Autodesk Inventor part; units mm, degrees
(part 2 of 2)
  line L284 (-20.2182, -37.2019) -> (-20.2182, -36.6708)
  line L285 (-20.2182, -36.6708) -> (-19.576, -36.6708)
  line L286 (-19.576, -36.6708) -> (-19.576, -35.0579)
  line L287 (-19.576, -35.0579) -> (-20.2182, -35.0579)
  line L288 (-20.2182, -35.0579) -> (-20.2182, -34.5614)
  spline S239 degree 2 poles (-20.2182, -34.5614) (-20.0774, -34.5614) (-19.7983, -34.5244) (-19.7143, -34.4848) knots 0 0 0 1 2 2 2
  spline S240 degree 2 poles (-19.7143, -34.4848) (-19.6179, -34.4354) (-19.5093, -34.27) (-19.4994, -34.1465) knots 0 0 0 1 2 2 2
  line L289 (-19.4994, -34.1465) -> (-18.8325, -34.1465)
  line L290 (-18.8325, -34.1465) -> (-18.8325, -36.6708)
  line L291 (-18.8325, -36.6708) -> (-18.2051, -36.6708)
  line L292 (-18.2051, -36.6708) -> (-18.2051, -37.2019)
  spline S241 degree 2 poles (-15.4164, -36.1645) (-15.4164, -36.6461) (-16.0265, -37.2661) (-16.5601, -37.2661) knots 0 0 0 1 2 2 2
  spline S242 degree 2 poles (-16.5601, -37.2661) (-16.8268, -37.2661) (-17.2443, -37.1129) (-17.39, -36.9623) knots 0 0 0 1 2 2 2
  spline S243 degree 2 poles (-17.39, -36.9623) (-17.5629, -36.7869) (-17.7481, -36.2312) (-17.7481, -35.8434) knots 0 0 0 1 2 2 2
  spline S244 degree 2 poles (-17.7481, -35.8434) (-17.7481, -35.4432) (-17.5752, -34.8208) (-17.3801, -34.5812) knots 0 0 0 1 2 2 2
  spline S245 degree 2 poles (-17.3801, -34.5812) (-17.1949, -34.3539) (-16.5922, -34.0971) (-16.1797, -34.0971) knots 0 0 0 1 2 2 2
  spline S246 degree 2 poles (-16.1797, -34.0971) (-16.029, -34.0971) (-15.7277, -34.1366) (-15.6733, -34.1489) knots 0 0 0 1 2 2 2
  line L293 (-15.6733, -34.1489) -> (-15.6733, -34.7467)
  line L294 (-15.6733, -34.7467) -> (-15.7277, -34.7467)
  spline S247 degree 2 poles (-15.7277, -34.7467) (-15.782, -34.7195) (-16.029, -34.6528) (-16.1871, -34.6528) knots 0 0 0 1 2 2 2
  spline S248 degree 2 poles (-16.1871, -34.6528) (-16.5452, -34.6528) (-16.9355, -35.0307) (-16.9824, -35.3815) knots 0 0 0 1 2 2 2
  spline S249 degree 2 poles (-16.9824, -35.3815) (-16.8318, -35.2851) (-16.523, -35.1715) (-16.3279, -35.1715) knots 0 0 0 1 2 2 2
  spline S250 degree 2 poles (-16.3279, -35.1715) (-16.1624, -35.1715) (-15.8734, -35.2604) (-15.7623, -35.3444) knots 0 0 0 1 2 2 2
  spline S251 degree 2 poles (-15.7623, -35.3444) (-15.6042, -35.4654) (-15.4164, -35.8582) (-15.4164, -36.1645) knots 0 0 0 1 2 2 2
  spline S252 degree 2 poles (-16.3081, -36.6239) (-16.2488, -36.5498) (-16.1846, -36.3769) (-16.1846, -36.2015) knots 0 0 0 1 2 2 2
  spline S253 degree 2 poles (-16.1846, -36.2015) (-16.1846, -36.0533) (-16.2587, -35.8606) (-16.3254, -35.8038) knots 0 0 0 1 2 2 2
  spline S254 degree 2 poles (-16.3254, -35.8038) (-16.3946, -35.7446) (-16.565, -35.7026) (-16.6613, -35.7026) knots 0 0 0 1 2 2 2
  spline S255 degree 2 poles (-16.6613, -35.7026) (-16.7428, -35.7026) (-16.9108, -35.7446) (-16.9849, -35.7742) knots 0 0 0 1 2 2 2
  spline S256 degree 2 poles (-16.9849, -35.7742) (-16.9849, -35.794) (-16.9899, -35.8878) (-16.9899, -35.9594) knots 0 0 0 1 2 2 2
  spline S257 degree 2 poles (-16.9899, -35.9594) (-16.9899, -36.2237) (-16.8985, -36.5424) (-16.8268, -36.6239) knots 0 0 0 1 2 2 2
  spline S258 degree 2 poles (-16.8268, -36.6239) (-16.775, -36.6906) (-16.6366, -36.7474) (-16.5625, -36.7474) knots 0 0 0 1 2 2 2
  spline S259 degree 2 poles (-16.5625, -36.7474) (-16.5008, -36.7474) (-16.3575, -36.6856) (-16.3081, -36.6239) knots 0 0 0 1 2 2 2
  line L295 (-13.0601, -37.2019) -> (-13.7764, -37.2019)
  line L296 (-13.7764, -37.2019) -> (-13.7764, -34.9023)
  line L297 (-13.7764, -34.9023) -> (-13.0601, -34.9023)
  line L298 (-13.0601, -34.9023) -> (-13.0601, -37.2019)
  line L299 (-13.0378, -34.5738) -> (-13.7961, -34.5738)
  line L300 (-13.7961, -34.5738) -> (-13.7961, -34.0155)
  line L301 (-13.7961, -34.0155) -> (-13.0378, -34.0155)
  line L302 (-13.0378, -34.0155) -> (-13.0378, -34.5738)
  line L303 (-10.3603, -37.2019) -> (-11.0816, -37.2019)
  line L304 (-11.0816, -37.2019) -> (-11.0816, -36.0632)
  spline S260 degree 2 poles (-11.0816, -36.0632) (-11.0816, -35.9224) (-11.1038, -35.6458) (-11.1334, -35.5815) knots 0 0 0 1 2 2 2
  spline S261 degree 2 poles (-11.1334, -35.5815) (-11.1705, -35.5025) (-11.3088, -35.4358) (-11.4274, -35.4358) knots 0 0 0 1 2 2 2
  spline S262 degree 2 poles (-11.4274, -35.4358) (-11.5138, -35.4358) (-11.6941, -35.5025) (-11.7954, -35.5741) knots 0 0 0 1 2 2 2
  line L305 (-11.7954, -35.5741) -> (-11.7954, -37.2019)
  line L306 (-11.7954, -37.2019) -> (-12.5117, -37.2019)
  line L307 (-12.5117, -37.2019) -> (-12.5117, -34.9023)
  line L308 (-12.5117, -34.9023) -> (-11.7954, -34.9023)
  line L309 (-11.7954, -34.9023) -> (-11.7954, -35.1567)
  spline S263 degree 2 poles (-11.7954, -35.1567) (-11.62, -35.0085) (-11.2866, -34.8405) (-11.084, -34.8405) knots 0 0 0 1 2 2 2
  spline S264 degree 2 poles (-11.084, -34.8405) (-10.7333, -34.8405) (-10.3603, -35.2851) (-10.3603, -35.705) knots 0 0 0 1 2 2 2
  line L310 (-10.3603, -35.705) -> (-10.3603, -37.2019)
  spline S265 degree 2 poles (-8.7029, -37.2636) (-8.987, -37.2636) (-9.4588, -37.1204) (-9.6341, -36.9722) knots 0 0 0 1 2 2 2
  spline S266 degree 2 poles (-9.6341, -36.9722) (-9.8046, -36.8215) (-9.9972, -36.3695) (-9.9972, -36.0632) knots 0 0 0 1 2 2 2
  spline S267 degree 2 poles (-9.9972, -36.0632) (-9.9972, -35.7322) (-9.7898, -35.2703) (-9.6094, -35.1221) knots 0 0 0 1 2 2 2
  spline S268 degree 2 poles (-9.6094, -35.1221) (-9.439, -34.9789) (-8.9746, -34.8405) (-8.7227, -34.8405) knots 0 0 0 1 2 2 2
  spline S269 degree 2 poles (-8.7227, -34.8405) (-8.5325, -34.8405) (-8.1521, -34.9295) (-7.9595, -35.0258) knots 0 0 0 1 2 2 2
  line L311 (-7.9595, -35.0258) -> (-7.9595, -35.6383)
  line L312 (-7.9595, -35.6383) -> (-8.0509, -35.6383)
  spline S270 degree 2 poles (-8.0509, -35.6383) (-8.0953, -35.5964) (-8.2188, -35.4976) (-8.2929, -35.458) knots 0 0 0 1 2 2 2
  spline S271 degree 2 poles (-8.2929, -35.458) (-8.372, -35.4136) (-8.5671, -35.3543) (-8.6881, -35.3543) knots 0 0 0 1 2 2 2
  spline S272 degree 2 poles (-8.6881, -35.3543) (-8.9623, -35.3543) (-9.2636, -35.7371) (-9.2636, -36.0632) knots 0 0 0 1 2 2 2
  spline S273 degree 2 poles (-9.2636, -36.0632) (-9.2636, -36.409) (-8.9425, -36.7499) (-8.6758, -36.7499) knots 0 0 0 1 2 2 2
  spline S274 degree 2 poles (-8.6758, -36.7499) (-8.5399, -36.7499) (-8.3374, -36.6881) (-8.2633, -36.6436) knots 0 0 0 1 2 2 2
  spline S275 degree 2 poles (-8.2633, -36.6436) (-8.1917, -36.6017) (-8.0879, -36.5078) (-8.0509, -36.4707) knots 0 0 0 1 2 2 2
  line L313 (-8.0509, -36.4707) -> (-7.9595, -36.4707)
  line L314 (-7.9595, -36.4707) -> (-7.9595, -37.0858)
  spline S276 degree 2 poles (-7.9595, -37.0858) (-8.0212, -37.1129) (-8.1818, -37.1821) (-8.2658, -37.2043) knots 0 0 0 1 2 2 2
  spline S277 degree 2 poles (-8.2658, -37.2043) (-8.3695, -37.234) (-8.5523, -37.2636) (-8.7029, -37.2636) knots 0 0 0 1 2 2 2
  line L315 (-5.4672, -37.2019) -> (-6.1885, -37.2019)
  line L316 (-6.1885, -37.2019) -> (-6.1885, -36.0632)
  spline S278 degree 2 poles (-6.1885, -36.0632) (-6.1885, -35.9224) (-6.2107, -35.6458) (-6.2403, -35.5815) knots 0 0 0 1 2 2 2
  spline S279 degree 2 poles (-6.2403, -35.5815) (-6.2774, -35.5025) (-6.4157, -35.4358) (-6.5343, -35.4358) knots 0 0 0 1 2 2 2
  spline S280 degree 2 poles (-6.5343, -35.4358) (-6.6207, -35.4358) (-6.801, -35.5025) (-6.9023, -35.5741) knots 0 0 0 1 2 2 2
  line L317 (-6.9023, -35.5741) -> (-6.9023, -37.2019)
  line L318 (-6.9023, -37.2019) -> (-7.6186, -37.2019)
  line L319 (-7.6186, -37.2019) -> (-7.6186, -34.018)
  line L320 (-7.6186, -34.018) -> (-6.9023, -34.018)
  line L321 (-6.9023, -34.018) -> (-6.9023, -35.1567)
  spline S281 degree 2 poles (-6.9023, -35.1567) (-6.7269, -35.0085) (-6.3935, -34.8405) (-6.1909, -34.8405) knots 0 0 0 1 2 2 2
  spline S282 degree 2 poles (-6.1909, -34.8405) (-5.8402, -34.8405) (-5.4672, -35.2851) (-5.4672, -35.705) knots 0 0 0 1 2 2 2
  line L322 (-5.4672, -35.705) -> (-5.4672, -37.2019)
  line L323 (6.2592, -34.759) -> (4.9575, -37.2019)
  line L324 (4.9575, -37.2019) -> (4.1078, -37.2019)
  line L325 (4.1078, -37.2019) -> (5.4687, -34.7294)
  line L326 (5.4687, -34.7294) -> (4.0164, -34.7294)
  line L327 (4.0164, -34.7294) -> (4.0164, -34.1539)
  line L328 (4.0164, -34.1539) -> (6.2592, -34.1539)
  line L329 (6.2592, -34.1539) -> (6.2592, -34.759)
  line L330 (8.4896, -34.018) -> (7.2768, -37.8638)
  line L331 (7.2768, -37.8638) -> (6.6889, -37.8638)
  line L332 (6.6889, -37.8638) -> (7.8992, -34.018)
  line L333 (7.8992, -34.018) -> (8.4896, -34.018)
  spline S283 degree 2 poles (11.3968, -36.1645) (11.3968, -36.6461) (10.7867, -37.2661) (10.2532, -37.2661) knots 0 0 0 1 2 2 2
  spline S284 degree 2 poles (10.2532, -37.2661) (9.9864, -37.2661) (9.569, -37.1129) (9.4232, -36.9623) knots 0 0 0 1 2 2 2
  spline S285 degree 2 poles (9.4232, -36.9623) (9.2503, -36.7869) (9.0651, -36.2312) (9.0651, -35.8434) knots 0 0 0 1 2 2 2
  spline S286 degree 2 poles (9.0651, -35.8434) (9.0651, -35.4432) (9.238, -34.8208) (9.4331, -34.5812) knots 0 0 0 1 2 2 2
  spline S287 degree 2 poles (9.4331, -34.5812) (9.6184, -34.3539) (10.2211, -34.0971) (10.6336, -34.0971) knots 0 0 0 1 2 2 2
  spline S288 degree 2 poles (10.6336, -34.0971) (10.7842, -34.0971) (11.0856, -34.1366) (11.1399, -34.1489) knots 0 0 0 1 2 2 2
  line L334 (11.1399, -34.1489) -> (11.1399, -34.7467)
  line L335 (11.1399, -34.7467) -> (11.0856, -34.7467)
  spline S289 degree 2 poles (11.0856, -34.7467) (11.0312, -34.7195) (10.7842, -34.6528) (10.6261, -34.6528) knots 0 0 0 1 2 2 2
  spline S290 degree 2 poles (10.6261, -34.6528) (10.268, -34.6528) (9.8777, -35.0307) (9.8308, -35.3815) knots 0 0 0 1 2 2 2
  spline S291 degree 2 poles (9.8308, -35.3815) (9.9815, -35.2851) (10.2902, -35.1715) (10.4854, -35.1715) knots 0 0 0 1 2 2 2
  spline S292 degree 2 poles (10.4854, -35.1715) (10.6508, -35.1715) (10.9398, -35.2604) (11.051, -35.3444) knots 0 0 0 1 2 2 2
  spline S293 degree 2 poles (11.051, -35.3444) (11.2091, -35.4654) (11.3968, -35.8582) (11.3968, -36.1645) knots 0 0 0 1 2 2 2
  spline S294 degree 2 poles (10.5051, -36.6239) (10.5644, -36.5498) (10.6286, -36.3769) (10.6286, -36.2015) knots 0 0 0 1 2 2 2
  spline S295 degree 2 poles (10.6286, -36.2015) (10.6286, -36.0533) (10.5545, -35.8606) (10.4878, -35.8038) knots 0 0 0 1 2 2 2
  spline S296 degree 2 poles (10.4878, -35.8038) (10.4187, -35.7446) (10.2482, -35.7026) (10.1519, -35.7026) knots 0 0 0 1 2 2 2
  spline S297 degree 2 poles (10.1519, -35.7026) (10.0704, -35.7026) (9.9024, -35.7446) (9.8283, -35.7742) knots 0 0 0 1 2 2 2
  spline S298 degree 2 poles (9.8283, -35.7742) (9.8283, -35.794) (9.8234, -35.8878) (9.8234, -35.9594) knots 0 0 0 1 2 2 2
  spline S299 degree 2 poles (9.8234, -35.9594) (9.8234, -36.2237) (9.9148, -36.5424) (9.9864, -36.6239) knots 0 0 0 1 2 2 2
  spline S300 degree 2 poles (9.9864, -36.6239) (10.0383, -36.6906) (10.1766, -36.7474) (10.2507, -36.7474) knots 0 0 0 1 2 2 2
  spline S301 degree 2 poles (10.2507, -36.7474) (10.3124, -36.7474) (10.4557, -36.6856) (10.5051, -36.6239) knots 0 0 0 1 2 2 2
  line L336 (13.7532, -37.2019) -> (13.0369, -37.2019)
  line L337 (13.0369, -37.2019) -> (13.0369, -34.9023)
  line L338 (13.0369, -34.9023) -> (13.7532, -34.9023)
  line L339 (13.7532, -34.9023) -> (13.7532, -37.2019)
  line L340 (13.7754, -34.5738) -> (13.0171, -34.5738)
  line L341 (13.0171, -34.5738) -> (13.0171, -34.0155)
  line L342 (13.0171, -34.0155) -> (13.7754, -34.0155)
  line L343 (13.7754, -34.0155) -> (13.7754, -34.5738)
  line L344 (16.4529, -37.2019) -> (15.7317, -37.2019)
  line L345 (15.7317, -37.2019) -> (15.7317, -36.0632)
  spline S302 degree 2 poles (15.7317, -36.0632) (15.7317, -35.9224) (15.7094, -35.6458) (15.6798, -35.5815) knots 0 0 0 1 2 2 2
  spline S303 degree 2 poles (15.6798, -35.5815) (15.6427, -35.5025) (15.5044, -35.4358) (15.3859, -35.4358) knots 0 0 0 1 2 2 2
  spline S304 degree 2 poles (15.3859, -35.4358) (15.2994, -35.4358) (15.1191, -35.5025) (15.0178, -35.5741) knots 0 0 0 1 2 2 2
  line L346 (15.0178, -35.5741) -> (15.0178, -37.2019)
  line L347 (15.0178, -37.2019) -> (14.3015, -37.2019)
  line L348 (14.3015, -37.2019) -> (14.3015, -34.9023)
  line L349 (14.3015, -34.9023) -> (15.0178, -34.9023)
  line L350 (15.0178, -34.9023) -> (15.0178, -35.1567)
  spline S305 degree 2 poles (15.0178, -35.1567) (15.1932, -35.0085) (15.5267, -34.8405) (15.7292, -34.8405) knots 0 0 0 1 2 2 2
  spline S306 degree 2 poles (15.7292, -34.8405) (16.0799, -34.8405) (16.4529, -35.2851) (16.4529, -35.705) knots 0 0 0 1 2 2 2
  line L351 (16.4529, -35.705) -> (16.4529, -37.2019)
  spline S307 degree 2 poles (18.1103, -37.2636) (17.8262, -37.2636) (17.3545, -37.1204) (17.1791, -36.9722) knots 0 0 0 1 2 2 2
  spline S308 degree 2 poles (17.1791, -36.9722) (17.0087, -36.8215) (16.816, -36.3695) (16.816, -36.0632) knots 0 0 0 1 2 2 2
  spline S309 degree 2 poles (16.816, -36.0632) (16.816, -35.7322) (17.0235, -35.2703) (17.2038, -35.1221) knots 0 0 0 1 2 2 2
  spline S310 degree 2 poles (17.2038, -35.1221) (17.3742, -34.9789) (17.8386, -34.8405) (18.0905, -34.8405) knots 0 0 0 1 2 2 2
  spline S311 degree 2 poles (18.0905, -34.8405) (18.2807, -34.8405) (18.6611, -34.9295) (18.8538, -35.0258) knots 0 0 0 1 2 2 2
  line L352 (18.8538, -35.0258) -> (18.8538, -35.6383)
  line L353 (18.8538, -35.6383) -> (18.7624, -35.6383)
  spline S312 degree 2 poles (18.7624, -35.6383) (18.7179, -35.5964) (18.5944, -35.4976) (18.5203, -35.458) knots 0 0 0 1 2 2 2
  spline S313 degree 2 poles (18.5203, -35.458) (18.4413, -35.4136) (18.2461, -35.3543) (18.1251, -35.3543) knots 0 0 0 1 2 2 2
  spline S314 degree 2 poles (18.1251, -35.3543) (17.8509, -35.3543) (17.5496, -35.7371) (17.5496, -36.0632) knots 0 0 0 1 2 2 2
  spline S315 degree 2 poles (17.5496, -36.0632) (17.5496, -36.409) (17.8707, -36.7499) (18.1375, -36.7499) knots 0 0 0 1 2 2 2
  spline S316 degree 2 poles (18.1375, -36.7499) (18.2733, -36.7499) (18.4759, -36.6881) (18.55, -36.6436) knots 0 0 0 1 2 2 2
  spline S317 degree 2 poles (18.55, -36.6436) (18.6216, -36.6017) (18.7253, -36.5078) (18.7624, -36.4707) knots 0 0 0 1 2 2 2
  line L354 (18.7624, -36.4707) -> (18.8538, -36.4707)
  line L355 (18.8538, -36.4707) -> (18.8538, -37.0858)
  spline S318 degree 2 poles (18.8538, -37.0858) (18.792, -37.1129) (18.6315, -37.1821) (18.5475, -37.2043) knots 0 0 0 1 2 2 2
  spline S319 degree 2 poles (18.5475, -37.2043) (18.4437, -37.234) (18.261, -37.2636) (18.1103, -37.2636) knots 0 0 0 1 2 2 2
  line L356 (21.346, -37.2019) -> (20.6248, -37.2019)
  line L357 (20.6248, -37.2019) -> (20.6248, -36.0632)
  spline S320 degree 2 poles (20.6248, -36.0632) (20.6248, -35.9224) (20.6025, -35.6458) (20.5729, -35.5815) knots 0 0 0 1 2 2 2
  spline S321 degree 2 poles (20.5729, -35.5815) (20.5358, -35.5025) (20.3975, -35.4358) (20.279, -35.4358) knots 0 0 0 1 2 2 2
  spline S322 degree 2 poles (20.279, -35.4358) (20.1925, -35.4358) (20.0122, -35.5025) (19.9109, -35.5741) knots 0 0 0 1 2 2 2
  line L358 (19.9109, -35.5741) -> (19.9109, -37.2019)
  line L359 (19.9109, -37.2019) -> (19.1946, -37.2019)
  line L360 (19.1946, -37.2019) -> (19.1946, -34.018)
  line L361 (19.1946, -34.018) -> (19.9109, -34.018)
  line L362 (19.9109, -34.018) -> (19.9109, -35.1567)
  spline S323 degree 2 poles (19.9109, -35.1567) (20.0863, -35.0085) (20.4198, -34.8405) (20.6223, -34.8405) knots 0 0 0 1 2 2 2
  spline S324 degree 2 poles (20.6223, -34.8405) (20.973, -34.8405) (21.346, -35.2851) (21.346, -35.705) knots 0 0 0 1 2 2 2
  line L363 (21.346, -35.705) -> (21.346, -37.2019)
  spline S325 degree 2 poles (36.3026, -36.2781) (36.3026, -36.5029) (36.1371, -36.8709) (35.9765, -36.9993) knots 0 0 0 1 2 2 2
  spline S326 degree 2 poles (35.9765, -36.9993) (35.816, -37.1278) (35.3788, -37.2661) (35.0651, -37.2661) knots 0 0 0 1 2 2 2
  spline S327 degree 2 poles (35.0651, -37.2661) (34.7094, -37.2661) (34.2006, -37.1475) (34.04, -37.0734) knots 0 0 0 1 2 2 2
  line L364 (34.04, -37.0734) -> (34.04, -36.4115)
  line L365 (34.04, -36.4115) -> (34.1141, -36.4115)
  spline S328 degree 2 poles (34.1141, -36.4115) (34.2821, -36.5177) (34.7341, -36.6758) (34.9218, -36.6758) knots 0 0 0 1 2 2 2
  spline S329 degree 2 poles (34.9218, -36.6758) (35.033, -36.6758) (35.2923, -36.6362) (35.3812, -36.572) knots 0 0 0 1 2 2 2
  spline S330 degree 2 poles (35.3812, -36.572) (35.4504, -36.5201) (35.5344, -36.3695) (35.5344, -36.2336) knots 0 0 0 1 2 2 2
  spline S331 degree 2 poles (35.5344, -36.2336) (35.5344, -36.0978) (35.4158, -35.952) (35.317, -35.9175) knots 0 0 0 1 2 2 2
  spline S332 degree 2 poles (35.317, -35.9175) (35.2182, -35.8829) (34.944, -35.8755) (34.8378, -35.8755) knots 0 0 0 1 2 2 2
  line L366 (34.8378, -35.8755) -> (34.7069, -35.8755)
  line L367 (34.7069, -35.8755) -> (34.7069, -35.3395)
  line L368 (34.7069, -35.3395) -> (34.828, -35.3395)
  spline S333 degree 2 poles (34.828, -35.3395) (34.9663, -35.3395) (35.2009, -35.3148) (35.2824, -35.2777) knots 0 0 0 1 2 2 2
  spline S334 degree 2 poles (35.2824, -35.2777) (35.3639, -35.2382) (35.4553, -35.0999) (35.4553, -34.9813) knots 0 0 0 1 2 2 2
  spline S335 degree 2 poles (35.4553, -34.9813) (35.4553, -34.8875) (35.3689, -34.7714) (35.3071, -34.7393) knots 0 0 0 1 2 2 2
  spline S336 degree 2 poles (35.3071, -34.7393) (35.233, -34.7022) (35.0354, -34.6775) (34.9663, -34.6775) knots 0 0 0 1 2 2 2
  spline S337 degree 2 poles (34.9663, -34.6775) (34.8551, -34.6775) (34.6205, -34.7294) (34.5118, -34.7714) knots 0 0 0 1 2 2 2
  spline S338 degree 2 poles (34.5118, -34.7714) (34.4253, -34.8035) (34.2376, -34.9072) (34.1932, -34.9344) knots 0 0 0 1 2 2 2
  line L369 (34.1932, -34.9344) -> (34.1289, -34.9344)
  line L370 (34.1289, -34.9344) -> (34.1289, -34.2823)
  spline S339 degree 2 poles (34.1289, -34.2823) (34.287, -34.2156) (34.8205, -34.0896) (35.0997, -34.0896) knots 0 0 0 1 2 2 2
  spline S340 degree 2 poles (35.0997, -34.0896) (35.3714, -34.0896) (35.7715, -34.1835) (35.9123, -34.2749) knots 0 0 0 1 2 2 2
  spline S341 degree 2 poles (35.9123, -34.2749) (36.0679, -34.3712) (36.2235, -34.6676) (36.2235, -34.8529) knots 0 0 0 1 2 2 2
  spline S342 degree 2 poles (36.2235, -34.8529) (36.2235, -35.1147) (35.9222, -35.505) (35.6752, -35.5618) knots 0 0 0 1 2 2 2
  line L371 (35.6752, -35.5618) -> (35.6752, -35.5914)
  spline S343 degree 2 poles (35.6752, -35.5914) (35.7838, -35.6062) (35.9913, -35.6853) (36.0901, -35.7742) knots 0 0 0 1 2 2 2
  spline S344 degree 2 poles (36.0901, -35.7742) (36.1815, -35.8532) (36.3026, -36.1052) (36.3026, -36.2781) knots 0 0 0 1 2 2 2
  line L372 (38.5429, -34.018) -> (37.3301, -37.8638)
  line L373 (37.3301, -37.8638) -> (36.7422, -37.8638)
  line L374 (36.7422, -37.8638) -> (37.9525, -34.018)
  line L375 (37.9525, -34.018) -> (38.5429, -34.018)
  spline S345 degree 2 poles (41.4599, -36.3547) (41.4599, -36.5498) (41.2969, -36.8882) (41.1413, -37.0117) knots 0 0 0 1 2 2 2
  spline S346 degree 2 poles (41.1413, -37.0117) (40.9857, -37.1352) (40.5386, -37.2735) (40.2496, -37.2735) knots 0 0 0 1 2 2 2
  spline S347 degree 2 poles (40.2496, -37.2735) (39.9409, -37.2735) (39.479, -37.1327) (39.3308, -37.0117) knots 0 0 0 1 2 2 2
  spline S348 degree 2 poles (39.3308, -37.0117) (39.1851, -36.8906) (39.0467, -36.5621) (39.0467, -36.3794) knots 0 0 0 1 2 2 2
  spline S349 degree 2 poles (39.0467, -36.3794) (39.0467, -36.1175) (39.3357, -35.7693) (39.6099, -35.6532) knots 0 0 0 1 2 2 2
  line L376 (39.6099, -35.6532) -> (39.6099, -35.6408)
  spline S350 degree 2 poles (39.6099, -35.6408) (39.3407, -35.5099) (39.1283, -35.1369) (39.1283, -34.9072) knots 0 0 0 1 2 2 2
  spline S351 degree 2 poles (39.1283, -34.9072) (39.1283, -34.7393) (39.2765, -34.4453) (39.4222, -34.3292) knots 0 0 0 1 2 2 2
  spline S352 degree 2 poles (39.4222, -34.3292) (39.563, -34.2181) (39.9903, -34.0847) (40.257, -34.0847) knots 0 0 0 1 2 2 2
  spline S353 degree 2 poles (40.257, -34.0847) (40.5386, -34.0847) (40.9585, -34.2057) (41.0944, -34.3045) knots 0 0 0 1 2 2 2
  spline S354 degree 2 poles (41.0944, -34.3045) (41.2327, -34.4033) (41.3809, -34.6899) (41.3809, -34.8554) knots 0 0 0 1 2 2 2
  spline S355 degree 2 poles (41.3809, -34.8554) (41.3809, -35.0727) (41.129, -35.421) (40.8696, -35.542) knots 0 0 0 1 2 2 2
  line L377 (40.8696, -35.542) -> (40.8696, -35.5519)
  spline S356 degree 2 poles (40.8696, -35.5519) (41.1734, -35.6754) (41.4599, -36.0755) (41.4599, -36.3547) knots 0 0 0 1 2 2 2
  spline S357 degree 2 poles (40.7041, -36.3868) (40.7041, -36.2361) (40.5757, -36.078) (40.3682, -35.9767) knots 0 0 0 1 2 2 2
  spline S358 degree 2 poles (40.3682, -35.9767) (40.3089, -35.9496) (40.0841, -35.8631) (39.9977, -35.8261) knots 0 0 0 1 2 2 2
  spline S359 degree 2 poles (39.9977, -35.8261) (39.9187, -35.9051) (39.7927, -36.1422) (39.7927, -36.283) knots 0 0 0 1 2 2 2
  spline S360 degree 2 poles (39.7927, -36.283) (39.7927, -36.4954) (40.0644, -36.7499) (40.2842, -36.7499) knots 0 0 0 1 2 2 2
  spline S361 degree 2 poles (40.2842, -36.7499) (40.346, -36.7499) (40.4991, -36.7103) (40.5584, -36.6708) knots 0 0 0 1 2 2 2
  spline S362 degree 2 poles (40.5584, -36.6708) (40.6251, -36.6239) (40.7041, -36.4954) (40.7041, -36.3868) knots 0 0 0 1 2 2 2
  spline S363 degree 2 poles (40.6374, -34.9443) (40.6374, -34.7887) (40.4324, -34.6034) (40.257, -34.6034) knots 0 0 0 1 2 2 2
  spline S364 degree 2 poles (40.257, -34.6034) (40.0891, -34.6034) (39.8841, -34.7714) (39.8841, -34.8949) knots 0 0 0 1 2 2 2
  spline S365 degree 2 poles (39.8841, -34.8949) (39.8841, -35.0159) (40.0076, -35.1666) (40.1385, -35.2283) knots 0 0 0 1 2 2 2
  spline S366 degree 2 poles (40.1385, -35.2283) (40.1953, -35.258) (40.3534, -35.3197) (40.4843, -35.3691) knots 0 0 0 1 2 2 2
  spline S367 degree 2 poles (40.4843, -35.3691) (40.5633, -35.2654) (40.6374, -35.0702) (40.6374, -34.9443) knots 0 0 0 1 2 2 2
  line L378 (43.8065, -37.2019) -> (43.0902, -37.2019)
  line L379 (43.0902, -37.2019) -> (43.0902, -34.9023)
  line L380 (43.0902, -34.9023) -> (43.8065, -34.9023)
  line L381 (43.8065, -34.9023) -> (43.8065, -37.2019)
  line L382 (43.8287, -34.5738) -> (43.0704, -34.5738)
  line L383 (43.0704, -34.5738) -> (43.0704, -34.0155)
  line L384 (43.0704, -34.0155) -> (43.8287, -34.0155)
  line L385 (43.8287, -34.0155) -> (43.8287, -34.5738)
  line L386 (46.5062, -37.2019) -> (45.7849, -37.2019)
  line L387 (45.7849, -37.2019) -> (45.7849, -36.0632)
  spline S368 degree 2 poles (45.7849, -36.0632) (45.7849, -35.9224) (45.7627, -35.6458) (45.7331, -35.5815) knots 0 0 0 1 2 2 2
  spline S369 degree 2 poles (45.7331, -35.5815) (45.696, -35.5025) (45.5577, -35.4358) (45.4391, -35.4358) knots 0 0 0 1 2 2 2
  spline S370 degree 2 poles (45.4391, -35.4358) (45.3527, -35.4358) (45.1724, -35.5025) (45.0711, -35.5741) knots 0 0 0 1 2 2 2
  line L388 (45.0711, -35.5741) -> (45.0711, -37.2019)
  line L389 (45.0711, -37.2019) -> (44.3548, -37.2019)
  line L390 (44.3548, -37.2019) -> (44.3548, -34.9023)
  line L391 (44.3548, -34.9023) -> (45.0711, -34.9023)
  line L392 (45.0711, -34.9023) -> (45.0711, -35.1567)
  spline S371 degree 2 poles (45.0711, -35.1567) (45.2465, -35.0085) (45.5799, -34.8405) (45.7825, -34.8405) knots 0 0 0 1 2 2 2
  spline S372 degree 2 poles (45.7825, -34.8405) (46.1332, -34.8405) (46.5062, -35.2851) (46.5062, -35.705) knots 0 0 0 1 2 2 2
  line L393 (46.5062, -35.705) -> (46.5062, -37.2019)
  spline S373 degree 2 poles (48.1636, -37.2636) (47.8795, -37.2636) (47.4077, -37.1204) (47.2324, -36.9722) knots 0 0 0 1 2 2 2
  spline S374 degree 2 poles (47.2324, -36.9722) (47.0619, -36.8215) (46.8693, -36.3695) (46.8693, -36.0632) knots 0 0 0 1 2 2 2
  spline S375 degree 2 poles (46.8693, -36.0632) (46.8693, -35.7322) (47.0768, -35.2703) (47.2571, -35.1221) knots 0 0 0 1 2 2 2
  spline S376 degree 2 poles (47.2571, -35.1221) (47.4275, -34.9789) (47.8919, -34.8405) (48.1438, -34.8405) knots 0 0 0 1 2 2 2
  spline S377 degree 2 poles (48.1438, -34.8405) (48.334, -34.8405) (48.7144, -34.9295) (48.907, -35.0258) knots 0 0 0 1 2 2 2
  line L394 (48.907, -35.0258) -> (48.907, -35.6383)
  line L395 (48.907, -35.6383) -> (48.8157, -35.6383)
  spline S378 degree 2 poles (48.8157, -35.6383) (48.7712, -35.5964) (48.6477, -35.4976) (48.5736, -35.458) knots 0 0 0 1 2 2 2
  spline S379 degree 2 poles (48.5736, -35.458) (48.4946, -35.4136) (48.2994, -35.3543) (48.1784, -35.3543) knots 0 0 0 1 2 2 2
  spline S380 degree 2 poles (48.1784, -35.3543) (47.9042, -35.3543) (47.6029, -35.7371) (47.6029, -36.0632) knots 0 0 0 1 2 2 2
  spline S381 degree 2 poles (47.6029, -36.0632) (47.6029, -36.409) (47.924, -36.7499) (48.1907, -36.7499) knots 0 0 0 1 2 2 2
  spline S382 degree 2 poles (48.1907, -36.7499) (48.3266, -36.7499) (48.5291, -36.6881) (48.6032, -36.6436) knots 0 0 0 1 2 2 2
  spline S383 degree 2 poles (48.6032, -36.6436) (48.6749, -36.6017) (48.7786, -36.5078) (48.8157, -36.4707) knots 0 0 0 1 2 2 2
  line L396 (48.8157, -36.4707) -> (48.907, -36.4707)
  line L397 (48.907, -36.4707) -> (48.907, -37.0858)
  spline S384 degree 2 poles (48.907, -37.0858) (48.8453, -37.1129) (48.6847, -37.1821) (48.6008, -37.2043) knots 0 0 0 1 2 2 2
  spline S385 degree 2 poles (48.6008, -37.2043) (48.497, -37.234) (48.3142, -37.2636) (48.1636, -37.2636) knots 0 0 0 1 2 2 2
  line L398 (51.3993, -37.2019) -> (50.678, -37.2019)
  line L399 (50.678, -37.2019) -> (50.678, -36.0632)
  spline S386 degree 2 poles (50.678, -36.0632) (50.678, -35.9224) (50.6558, -35.6458) (50.6262, -35.5815) knots 0 0 0 1 2 2 2
  spline S387 degree 2 poles (50.6262, -35.5815) (50.5891, -35.5025) (50.4508, -35.4358) (50.3322, -35.4358) knots 0 0 0 1 2 2 2
  spline S388 degree 2 poles (50.3322, -35.4358) (50.2458, -35.4358) (50.0655, -35.5025) (49.9642, -35.5741) knots 0 0 0 1 2 2 2
  line L400 (49.9642, -35.5741) -> (49.9642, -37.2019)
  line L401 (49.9642, -37.2019) -> (49.2479, -37.2019)
  line L402 (49.2479, -37.2019) -> (49.2479, -34.018)
  line L403 (49.2479, -34.018) -> (49.9642, -34.018)
  line L404 (49.9642, -34.018) -> (49.9642, -35.1567)
  spline S389 degree 2 poles (49.9642, -35.1567) (50.1396, -35.0085) (50.473, -34.8405) (50.6756, -34.8405) knots 0 0 0 1 2 2 2
  spline S390 degree 2 poles (50.6756, -34.8405) (51.0263, -34.8405) (51.3993, -35.2851) (51.3993, -35.705) knots 0 0 0 1 2 2 2
  line L405 (51.3993, -35.705) -> (51.3993, -37.2019)
  point P0 (0, 0)
  dimension "d45" = 8.7721
  dimension "d46" = 40.64
  dimension "d50" = 90
  dimension "d52" = 90
  dimension "d53" = 90
  dimension "d54" = 90
  dimension "d55" = 90
  dimension "d56" = 90
  constraints: 48 end point, 15 horizontal, 14 point on circle, 7 parallel, 3 collinear, 3 tangent, 2 perpendicular, 2 vertical, 1 horizontal alignment, 1 other
  measures "d45" distance between parallel lines of L1 L0
  measures "d46" distance between parallel lines of L5 L0
  measures "d50" angle of L9 L2
  measures "d52" angle of L11 L1
  measures "d53" angle of L13 L3
  measures "d54" angle of L15 L4
  measures "d55" angle of L19 L6
  measures "d56" angle of L21 L7
extrude "textLabels" cut sketch "Sketch7" against normal blind 3.175
fillet "Fillet1" radius 3.175 8 edges at (-53.7972, 0, -12.7) (-27.8384, 0, -12.7) (1.9304, 0, -12.7) (31.4452, 0, -12.7) (35.6311, 0, 19.05) (6.4668, 0, 19.05) (-20.6654, 0, 19.05) (-46.7817, 0, 19.05)
fillet "Fillet2" radius 3.175 4 edges at (-63.5, -4.7625, 44.45) (-63.5, -4.7625, -44.45) (63.5, -4.7625, 44.45) (63.5, -4.7625, -44.45)
equation "\"gap0\" = frontGapBetweenHoles"
equation "\"gap1\" = 0.5 * hex5_16inchHole + 0.5 * hex1_4inchHole + frontGapBetweenHoles"
equation "\"gap2\" = 0.5 * hex3_8inchHole + 0.5 * hex5_16inchHole + frontGapBetweenHoles"
equation "\"gap3\" = 0.5 * hex7_16inchHole + 0.5 * hex3_8inchHole + frontGapBetweenHoles"
equation "\"gap5\" = backGapBetweenHoles"
equation "\"gap6\" = 0.5 * hex9_16inchHole + 0.5 * hex1_2inchHole + backGapBetweenHoles"
equation "\"gap7\" = 0.5 * hex5_8inchHole + 0.5 * hex9_16inchHole + backGapBetweenHoles"
equation "\"gap8\" = 0.5 * hex3_4inchHole + 0.5 * hex5_8inchHole + backGapBetweenHoles"
equation "\"d46\" = centerLineForBackText"
equation "\"frontGapBetweenHoles\" = 16.71828"
equation "\"backGapBetweenHoles\" = 9.7028"
equation "\"centerLineForFrontText\" = 8.3185"
equation "\"centerLineForBackText\" = 40.64"
body "Solid1"
